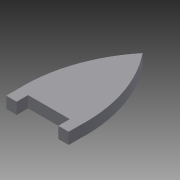
# Autodesk Inventor part: oreja
Saved by Autodesk Inventor 2015 (Build 190159000, 159)
## iProperties
Created: 2017-11-29
Part Number: oreja
Material: Generic
Document SubType Name: Modeling
Designer: Max
Density: 1 g/cm^3
Appearance: Default
Author: Max
Autodesk Inventor part; units mm, degrees
ref_plane "YZ Plane" through (0, 0, 0) normal (1, 0, 0) x (0, 1, 0)
ref_plane "XZ Plane" through (0, 0, 0) normal (0, 1, 0) x (-1, 0, 0)
ref_plane "XY Plane" through (0, 0, 0) normal (0, 0, 1) x (1, 0, 0)
sketch "Sketch1" plane through (0, 0, 0) normal (0, 0, 1) x (1, 0, 0)
  line L0 (0, 0) -> (-10, 0)
  arc A0 (0, 45) -> (-15, 0) centre (52.0178, 2.6607) ccw
  line L1 (-15, 0) -> (-15, -5.5)
  line L2 (-15, -5.5) -> (-10, -5.5)
  line L3 (-10, -5.5) -> (-10, 0)
  line L4 (0, 0) -> (10, 0)
  arc A1 (15, 0) -> (0, 45) centre (-52.0178, 2.6607) ccw
  line L5 (15, 0) -> (15, -5.5)
  line L6 (15, -5.5) -> (10, -5.5)
  line L7 (10, -5.5) -> (10, 0)
  dimension "d0" = 15
  dimension "d1" = 5.5
  dimension "d2" = 5
  constraints: 16 end point, 4 point on circle, 2 centre point, 2 perpendicular, 1 horizontal, 1 vertical
  measures "d0" distance of L0.start L1.start
  measures "d1" distance of L1.start L1.end
  measures "d2" distance of L1.end L2.end
extrude "Extrusion1" add sketch "Sketch1" along normal blind 5.5
body "Solid1"
